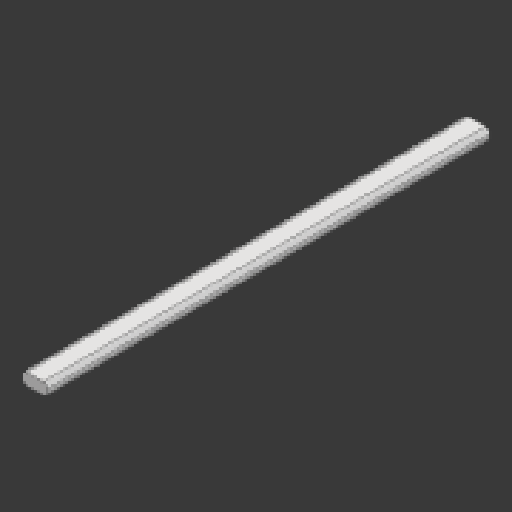
# Autodesk Inventor part: Led Light
Saved by Autodesk Inventor 2023 (Build 270158000, 158)
## iProperties
Created: 2023-01-04
Part Number: Led Light
Material: Generic
Document SubType Name: Modeling
Designer: alber
Density: 1 g/cm^3
Appearance: Default
Author: alber
Autodesk Inventor part; units mm, degrees
ref_plane "YZ Plane" through (0, 0, 0) normal (1, 0, 0) x (0, 1, 0)
ref_plane "XZ Plane" through (0, 0, 0) normal (0, 1, 0) x (-1, 0, 0)
ref_plane "XY Plane" through (0, 0, 0) normal (0, 0, 1) x (1, 0, 0)
sketch "Sketch1" plane through (0, 0, 0) normal (0, 1, 0) x (-1, 0, 0)
  line L0 (8.75, -154) -> (-8.75, -154)
  line L1 (-8.75, -154) -> (-8.75, 154)
  line L2 (-8.75, 154) -> (8.75, 154)
  line L3 (8.75, 154) -> (8.75, -154)
  line L4 (8.75, -154) -> (-8.75, 154) construction
  line L5 (-8.75, -154) -> (8.75, 154) construction
  point P0 (0, 0)
  dimension "d0" = 17.5
  dimension "d1" = 308
  constraints: 12 end point, 2 midpoint, 2 parallel, 1 horizontal, 1 perpendicular
  measures "d0" distance of L1.end L2.end
  measures "d1" distance of L0.end L1.end
extrude "Extrusion1" add sketch "Sketch1" along normal blind 8
fillet "Fillet1" radius 3 4 edges at (8.75, 8, 0) (-8.75, 8, 0) (-8.75, 0, 0) (8.75, 0, 0)
body "Solid1"
